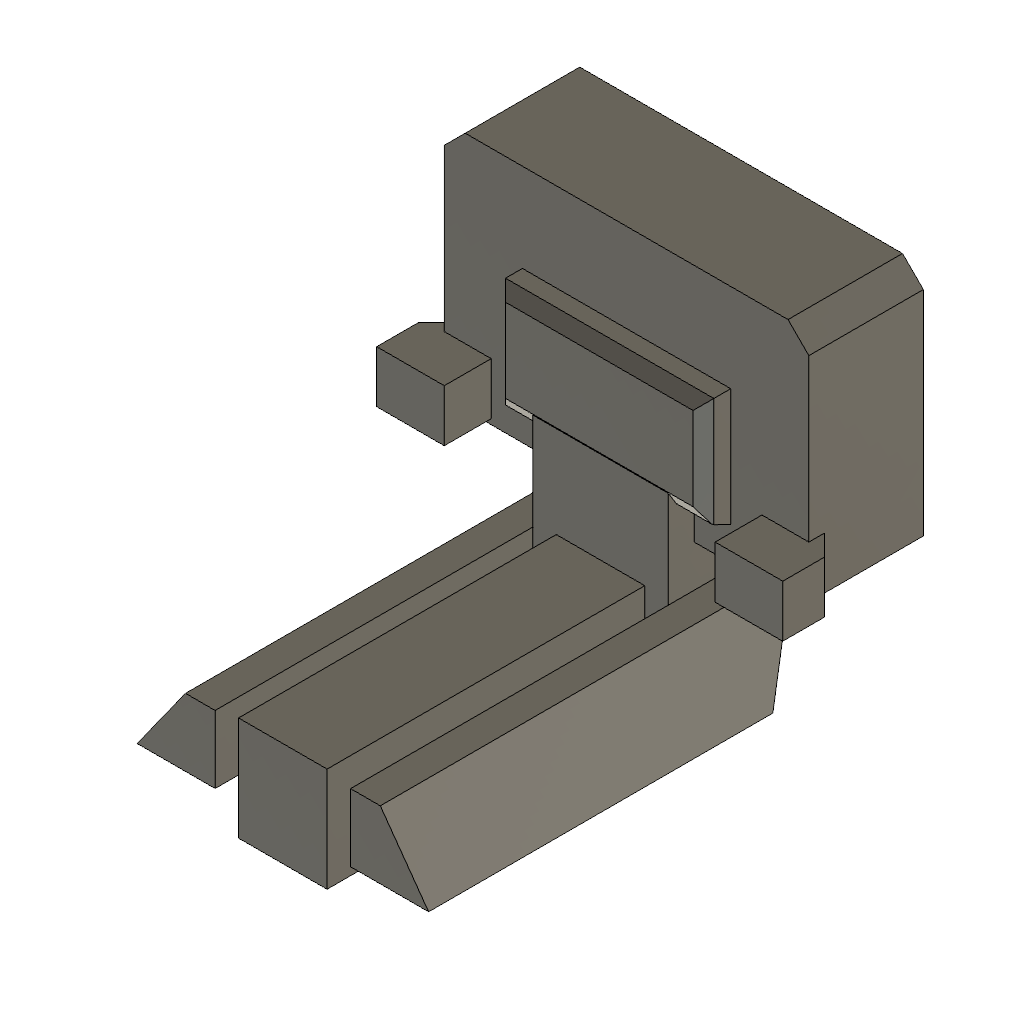
R9_G20_button_2_LEFT_USB (Autodesk Fusion 360 design; units mm, degrees)
part number: 2026-10-05-03-56-12-437
Autodesk Fusion 360 part; units mm, degrees
ref_plane "工作平面1" through (0, -32.4, 0) normal (0, 1, 0) x (0, 0, 1)
sketch "草图1" plane through (0, -32.4, 0) normal (0, 1, 0) x (1, 0, 0)
  line L0 (2.0205, 7.3, 64.8) -> (7.4205, 7.3, 64.8)
  line L1 (7.4205, 7.3, 64.8) -> (7.7205, 7, 64.8)
  line L2 (7.7205, 7, 64.8) -> (7.7205, 3.5, 64.8)
  line L3 (7.7205, 3.5, 64.8) -> (7.4205, 3.2, 64.8)
  line L4 (7.4205, 3.2, 64.8) -> (2.0205, 3.2, 64.8)
  line L5 (2.0205, 3.2, 64.8) -> (1.7205, 3.5, 64.8)
  line L6 (1.7205, 3.5, 64.8) -> (1.7205, 7, 64.8)
  line L7 (1.7205, 7, 64.8) -> (2.0205, 7.3, 64.8)
extrude "R6 rounded corner cap recessed 0.10mm" add sketch "草图1" along normal blind 2.2 contours L0 L1 L2 L3 L4 L5 L6 L7 in plane through (0, 32.4, 0) normal (0, 1, 0)
ref_plane "工作平面2" through (0, -31.9, 0) normal (0, 1, 0) x (0, 0, 1)
sketch "草图2" plane through (0, -31.9, 0) normal (0, 1, 0) x (1, 0, 0)
  line L0 (1.9205, 9.5, 63.8) -> (7.5205, 9.5, 63.8)
  line L1 (7.5205, 9.5, 63.8) -> (6.5205, 8.1, 63.8)
  line L2 (6.5205, 8.1, 63.8) -> (6.0205, 8.1, 63.8)
  line L3 (6.0205, 8.1, 63.8) -> (6.0205, 7.25, 63.8)
  line L4 (6.0205, 7.25, 63.8) -> (3.4205, 7.25, 63.8)
  line L5 (3.4205, 7.25, 63.8) -> (3.4205, 8.1, 63.8)
  line L6 (3.4205, 8.1, 63.8) -> (2.9205, 8.1, 63.8)
  line L7 (2.9205, 8.1, 63.8) -> (1.9205, 9.5, 63.8)
extrude "R6 track compatible dovetail neck" add sketch "草图2" along normal blind 2.7 contours L0 L1 L2 L3 L4 L5 L6 L7 in plane through (0, 31.9, 0) normal (0, 1, 0)
ref_plane "工作平面3" through (1.6205, 0, 0) normal (1, 0, 0) x (0, 1, 0)
sketch "草图3" plane through (1.6205, 0, 0) normal (1, 0, 0) x (0, 0, -1)
  line L0 (9.51, 32.4) -> (9.51, 34.61)
  line L1 (9.51, 34.61) -> (7.29, 34.61)
  line L2 (7.29, 34.61) -> (9.51, 32.4)
extrude "R6 45deg lower neck printing relief" cut sketch "草图3" along normal blind 6.2
ref_plane "工作平面4" through (0, -25.8, 0) normal (0, 1, 0) x (0, 0, 1)
sketch "草图4" plane through (0, -25.8, 0) normal (0, 1, 0) x (1, 0, 0)
  line L0 (3.4205, 9.5, 51.6) -> (1.9205, 9.5, 51.6)
  line L1 (1.9205, 9.5, 51.6) -> (2.9205, 8.1, 51.6)
  line L2 (2.9205, 8.1, 51.6) -> (3.4205, 8.1, 51.6)
  line L3 (3.4205, 8.1, 51.6) -> (3.4205, 9.5, 51.6)
extrude "R6 6.3mm guide runner -1" add sketch "草图4" along normal blind 6.3 contours L0 L1 L2 L3 in plane through (0, 25.8, 0) normal (0, 1, 0)
ref_plane "工作平面5" through (0, 0, -7.3) normal (0, 0, 1) x (1, 0, 0)
sketch "草图5" plane through (0, 0, -7.3) normal (0, 0, 1) x (1, 0, 0)
  line L0 (2.1205, 31.5) -> (0.8205, 31.5)
  line L1 (0.8205, 31.5) -> (0.8205, 32.3)
  line L2 (0.8205, 32.3) -> (1.7205, 33.2)
  line L3 (1.7205, 33.2) -> (2.1205, 33.2)
  line L4 (2.1205, 33.2) -> (2.1205, 31.5)
extrude "R6 shoulder above rail roof -1" add sketch "草图5" along normal blind 1
ref_plane "工作平面6" through (0, -25.8, 0) normal (0, 1, 0) x (0, 0, 1)
sketch "草图6" plane through (0, -25.8, 0) normal (0, 1, 0) x (1, 0, 0)
  line L0 (6.0205, 9.5, 51.6) -> (7.5205, 9.5, 51.6)
  line L1 (7.5205, 9.5, 51.6) -> (6.5205, 8.1, 51.6)
  line L2 (6.5205, 8.1, 51.6) -> (6.0205, 8.1, 51.6)
  line L3 (6.0205, 8.1, 51.6) -> (6.0205, 9.5, 51.6)
extrude "R6 6.3mm guide runner 1" add sketch "草图6" along normal blind 6.3 contours L0 L1 L2 L3 in plane through (0, 25.8, 0) normal (0, 1, 0)
ref_plane "工作平面7" through (0, 0, -7.3) normal (0, 0, 1) x (1, 0, 0)
sketch "草图7" plane through (0, 0, -7.3) normal (0, 0, 1) x (1, 0, 0)
  line L0 (7.3205, 31.5) -> (8.6205, 31.5)
  line L1 (8.6205, 31.5) -> (8.6205, 32.3)
  line L2 (8.6205, 32.3) -> (7.7205, 33.2)
  line L3 (7.7205, 33.2) -> (7.3205, 33.2)
  line L4 (7.3205, 33.2) -> (7.3205, 31.5)
extrude "R6 shoulder above rail roof 1" add sketch "草图7" along normal blind 1
ref_plane "工作平面8" through (0, 0, -9.1) normal (0, 0, 1) x (1, 0, 0)
sketch "草图8" plane through (0, 0, -9.1) normal (0, 0, 1) x (1, 0, 0)
  line L0 (3.8705, 25.8) -> (5.5705, 25.8)
  line L1 (5.5705, 25.8) -> (5.5705, 32.05)
  line L2 (5.5705, 32.05) -> (3.8705, 32.05)
  line L3 (3.8705, 32.05) -> (3.8705, 25.8)
extrude "R6 1mm assembly latch leaf" add sketch "草图8" along normal blind 1
ref_plane "工作平面9" through (3.8705, 0, 0) normal (1, 0, 0) x (0, 1, 0)
sketch "草图9" plane through (3.8705, 0, 0) normal (1, 0, 0) x (0, 0, -1)
  line L0 (10.1, 25.8) -> (10.1, 26.4)
  line L1 (10.1, 26.4) -> (9.1, 27.4)
  line L2 (9.1, 27.4) -> (9.1, 25.8)
  line L3 (9.1, 25.8) -> (10.1, 25.8)
extrude "R6 45deg latch ramp" add sketch "草图9" along normal blind 1.7
ref_plane "工作平面10" through (3.8205, 0, 0) normal (1, 0, 0) x (0, 1, 0)
sketch "草图10" plane through (3.8205, 0, 0) normal (1, 0, 0) x (0, 0, -1)
  line L0 (7.3, 33.5) -> (4.9, 33.5)
  line L1 (4.9, 33.5) -> (4.9, 31.876)
  line L2 (4.9, 31.876) -> (6.1, 31.876)
  line L3 (6.1, 31.876) -> (7.3, 33.5)
extrude "R6 centered switch contact" add sketch "草图10" along normal blind 1.8
ref_plane "工作平面11" through (0, 0, -7.5) normal (0, 0, 1) x (1, 0, 0)
sketch "草图11" plane through (0, 0, -7.5) normal (0, 0, 1) x (1, 0, 0)
  line L0 (3.4105, 31.89) -> (6.0305, 31.89)
  line L1 (6.0305, 31.89) -> (6.0305, 32.39)
  line L2 (6.0305, 32.39) -> (3.4105, 32.39)
  line L3 (3.4105, 32.39) -> (3.4105, 31.89)
extrude "R6 rear neck switch body clearance 2" cut sketch "草图11" along normal blind 0.26
ref_plane "工作平面12" through (0, 0, -8.2) normal (0, 0, 1) x (1, 0, 0)
sketch "草图12" plane through (0, 0, -8.2) normal (0, 0, 1) x (1, 0, 0)
  line L0 (1.7105, 25.79) -> (3.4205, 25.79)
  line L1 (3.4205, 25.79) -> (3.4205, 34.39)
  line L2 (3.4205, 34.39) -> (1.7105, 34.39)
  line L3 (1.7105, 34.39) -> (1.7105, 25.79)
extrude "R6 guide vertical 0.35mm clearance 2 -1" cut sketch "草图12" along normal blind 0.11
ref_plane "工作平面13" through (0, 0, -8.2) normal (0, 0, 1) x (1, 0, 0)
sketch "草图13" plane through (0, 0, -8.2) normal (0, 0, 1) x (1, 0, 0)
  line L0 (6.0205, 25.79) -> (7.7305, 25.79)
  line L1 (7.7305, 25.79) -> (7.7305, 34.39)
  line L2 (7.7305, 34.39) -> (6.0205, 34.39)
  line L3 (6.0205, 34.39) -> (6.0205, 25.79)
extrude "R6 guide vertical 0.35mm clearance 2 1" cut sketch "草图13" along normal blind 0.11
ref_plane "工作平面14" through (0, -32.4, 0) normal (0, 1, 0) x (0, 0, 1)
sketch "草图14" plane through (0, -32.4, 0) normal (0, 1, 0) x (1, 0, 0)
  line L0 (1.7705, 7.6, 64.8) -> (7.6705, 7.6, 64.8)
  line L1 (7.6705, 7.6, 64.8) -> (8.0205, 7.25, 64.8)
  line L2 (8.0205, 7.25, 64.8) -> (8.0205, 3.25, 64.8)
  line L3 (8.0205, 3.25, 64.8) -> (7.6705, 2.9, 64.8)
  line L4 (7.6705, 2.9, 64.8) -> (1.7705, 2.9, 64.8)
  line L5 (1.7705, 2.9, 64.8) -> (1.4205, 3.25, 64.8)
  line L6 (1.4205, 3.25, 64.8) -> (1.4205, 7.25, 64.8)
  line L7 (1.4205, 7.25, 64.8) -> (1.7705, 7.6, 64.8)
extrude "R7A cap 6.60 x 4.70 mm - unchanged 0.10 recess" add sketch "草图14" along normal blind 2.2 contours L0 L1 L2 L3 L4 L5 L6 L7 in plane through (0, 32.4, 0) normal (0, 1, 0)
ref_plane "工作平面15" through (0, -26.1, 0) normal (0, 1, 0) x (0, 0, 1)
sketch "草图15" plane through (0, -26.1, 0) normal (0, 1, 0) x (1, 0, 0)
  line L0 (3.4205, 9.5, 52.2) -> (1.8205, 9.5, 52.2)
  line L1 (1.8205, 9.5, 52.2) -> (2.8205, 8.1, 52.2)
  line L2 (2.8205, 8.1, 52.2) -> (3.4205, 8.1, 52.2)
  line L3 (3.4205, 8.1, 52.2) -> (3.4205, 9.5, 52.2)
ref_plane "工作平面16" through (0, -26.1, 0) normal (0, 1, 0) x (0, 0, 1)
sketch "草图16" plane through (0, -26.1, 0) normal (0, 1, 0) x (1, 0, 0)
  line L0 (6.0205, 9.5, 52.2) -> (7.6205, 9.5, 52.2)
  line L1 (7.6205, 9.5, 52.2) -> (6.6205, 8.1, 52.2)
  line L2 (6.6205, 8.1, 52.2) -> (6.0205, 8.1, 52.2)
  line L3 (6.0205, 8.1, 52.2) -> (6.0205, 9.5, 52.2)
ref_plane "工作平面17" through (0, -32.4, 0) normal (0, 1, 0) x (0, 0, 1)
sketch "草图17" plane through (0, -32.4, 0) normal (0, 1, 0) x (1, 0, 0)
  line L0 (1.7205, 7.6, 64.8) -> (7.7205, 7.6, 64.8)
  line L1 (7.7205, 7.6, 64.8) -> (8.1205, 7.2, 64.8)
  line L2 (8.1205, 7.2, 64.8) -> (8.1205, 3.3, 64.8)
  line L3 (8.1205, 3.3, 64.8) -> (7.7205, 2.9, 64.8)
  line L4 (7.7205, 2.9, 64.8) -> (1.7205, 2.9, 64.8)
  line L5 (1.7205, 2.9, 64.8) -> (1.3205, 3.3, 64.8)
  line L6 (1.3205, 3.3, 64.8) -> (1.3205, 7.2, 64.8)
  line L7 (1.3205, 7.2, 64.8) -> (1.7205, 7.6, 64.8)
extrude "R8 visible cap 6.8x4.7 separate from 0.35 guide" add sketch "草图17" along normal blind 2.2 contours L0 L1 L2 L3 L4 L5 L6 L7 in plane through (0, 32.4, 0) normal (0, 1, 0)
ref_plane "工作平面18" through (0, 0, -7.4) normal (0, 0, 1) x (1, 0, 0)
sketch "草图18" plane through (0, 0, -7.4) normal (0, 0, 1) x (1, 0, 0)
  line L0 (3.7105, 30) -> (5.7305, 30)
  line L1 (5.7305, 30) -> (5.7305, 32.4001)
  line L2 (5.7305, 32.4001) -> (3.7105, 32.4001)
  line L3 (3.7105, 32.4001) -> (3.7105, 30)
extrude "R8 remove old narrow contact nose" cut sketch "草图18" along normal blind 2.6
ref_plane "工作平面19" through (2.7205, 0, 0) normal (1, 0, 0) x (0, 1, 0)
sketch "草图19" plane through (2.7205, 0, 0) normal (1, 0, 0) x (0, 0, -1)
  line L0 (7.3, 33.5) -> (4.5, 33.5)
  line L1 (4.5, 33.5) -> (4.5, 31.876)
  line L2 (4.5, 31.876) -> (6.5, 31.876)
  line L3 (6.5, 31.876) -> (7.3, 33.5)
extrude "R8 broad centered contact 4x2 G20" add sketch "草图19" along normal blind 4
chamfer "倒角1" distance 0.2 angle 45 4 edges at (4.7205, 31.876, -6.5) (2.7205, 31.876, -5.5) (6.7205, 31.876, -5.5) (4.7205, 31.876, -4.5) tangent chain off
ref_plane "工作平面20" through (0, -32.4, 0) normal (0, 1, 0) x (0, 0, 1)
sketch "草图20" plane through (0, -32.4, 0) normal (0, 1, 0) x (1, 0, 0)
  line L0 (1.7205, 7.7, 64.8) -> (7.7205, 7.7, 64.8)
  line L1 (7.7205, 7.7, 64.8) -> (8.1205, 7.3, 64.8)
  line L2 (8.1205, 7.3, 64.8) -> (8.1205, 3.2, 64.8)
  line L3 (8.1205, 3.2, 64.8) -> (7.7205, 2.8, 64.8)
  line L4 (7.7205, 2.8, 64.8) -> (1.7205, 2.8, 64.8)
  line L5 (1.7205, 2.8, 64.8) -> (1.3205, 3.2, 64.8)
  line L6 (1.3205, 3.2, 64.8) -> (1.3205, 7.3, 64.8)
  line L7 (1.3205, 7.3, 64.8) -> (1.7205, 7.7, 64.8)
extrude "R8 FINAL cap 6.8x4.9 - four straight edge gaps 0.20" add sketch "草图20" along normal blind 2.2 contours L0 L1 L2 L3 L4 L5 L6 L7 in plane through (0, 32.4, 0) normal (0, 1, 0)
ref_plane "工作平面21" through (1.2205, 0, 0) normal (1, 0, 0) x (0, 1, 0)
sketch "草图21" plane through (1.2205, 0, 0) normal (1, 0, 0) x (0, 0, -1)
  line L0 (7.71, 32.39) -> (7.71, 34)
  line L1 (7.71, 34) -> (7.4, 33.69)
  line L2 (7.4, 33.69) -> (7.4, 32.39)
  line L3 (7.4, 32.39) -> (7.71, 32.39)
extrude "R8 rear underside assembly relief - full visible cap retained" cut sketch "草图21" along normal blind 7
ref_plane "工作平面22" through (0, -32.4, 0) normal (0, 1, 0) x (0, 0, 1)
sketch "草图22" plane through (0, -32.4, 0) normal (0, 1, 0) x (1, 0, 0)
  line L0 (1.6205, 7.7, 64.8) -> (7.8205, 7.7, 64.8)
  line L1 (7.8205, 7.7, 64.8) -> (8.2205, 7.3, 64.8)
  line L2 (8.2205, 7.3, 64.8) -> (8.2205, 3.2, 64.8)
  line L3 (8.2205, 3.2, 64.8) -> (7.8205, 2.8, 64.8)
  line L4 (7.8205, 2.8, 64.8) -> (1.6205, 2.8, 64.8)
  line L5 (1.6205, 2.8, 64.8) -> (1.2205, 3.2, 64.8)
  line L6 (1.2205, 3.2, 64.8) -> (1.2205, 7.3, 64.8)
  line L7 (1.2205, 7.3, 64.8) -> (1.6205, 7.7, 64.8)
extrude "R9 visible cap WIDTH 7.0 HEIGHT unchanged 4.9" add sketch "草图22" along normal blind 2.2 contours L0 L1 L2 L3 L4 L5 L6 L7 in plane through (0, 32.4, 0) normal (0, 1, 0)
ref_plane "工作平面23" through (1.1205, 0, 0) normal (1, 0, 0) x (0, 1, 0)
sketch "草图23" plane through (1.1205, 0, 0) normal (1, 0, 0) x (0, 0, -1)
  line L0 (7.71, 32.39) -> (7.71, 34)
  line L1 (7.71, 34) -> (7.4, 33.69)
  line L2 (7.4, 33.69) -> (7.4, 32.39)
  line L3 (7.4, 32.39) -> (7.71, 32.39)
extrude "R9 preserve hidden outer assembly relief" cut sketch "草图23" along normal blind 7.2
ref_plane "工作平面24" through (0, 0, -8.1) normal (0, 0, 1) x (1, 0, 0)
sketch "草图24" plane through (0, 0, -8.1) normal (0, 0, 1) x (1, 0, 0)
  line L0 (3.4205, 31.9) -> (6.0205, 31.9)
  line L1 (6.0205, 31.9) -> (6.0205, 33.5)
  line L2 (6.0205, 33.5) -> (3.4205, 33.5)
  line L3 (3.4205, 33.5) -> (3.4205, 31.9)
extrude "R9 central connection web 2.6 wide x 1.8 high x 1.6 long" add sketch "草图24" along normal blind 1.8
